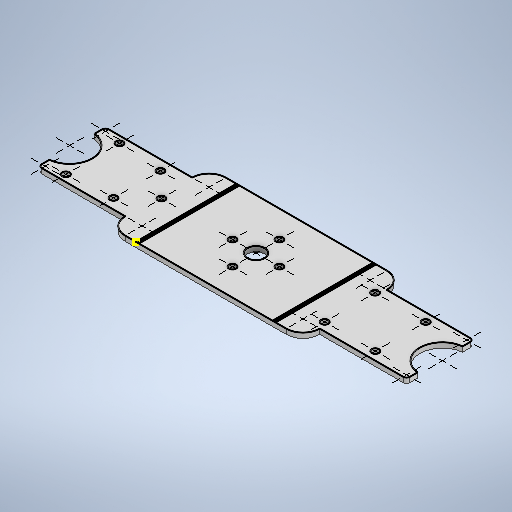
# Autodesk Inventor part: axis_13_top_frame
Saved by Autodesk Inventor 2026.1 (Build 301233000, 233)
## iProperties
Created: 2025-08-22
Part Number: axis_13_top_frame
Material: Generic
Document SubType Name: Modeling
Designer: LG
Density: 1 g/cm^3
Appearance: Default
Author: LG
Autodesk Inventor part; units mm, degrees
ref_plane "YZ Plane" through (0, 0, 0) normal (1, 0, 0) x (0, 1, 0)
ref_plane "XZ Plane" through (0, 0, 0) normal (0, 1, 0) x (-1, 0, 0)
ref_plane "XY Plane" through (0, 0, 0) normal (0, 0, 1) x (1, 0, 0)
sketch "Sketch1" plane through (0, 0, 0) normal (0, 1, 0) x (-1, 0, 0)
  line L0 (-0.4496, -30) -> (-0.4496, 0)
  line L1 (-41.2289, 0) -> (-41.2289, -30)
  circle A0 centre (-48.8686, -22.525) radius 1.05
  circle A1 centre (-48.8686, -7.475) radius 1.05
  circle A2 centre (-63.9686, -22.525) radius 1.05
  circle A3 centre (-63.9686, -7.475) radius 1.05
  circle A4 centre (27.89, -23) radius 1.05
  circle A5 centre (27.89, -7) radius 1.05
  circle A6 centre (14.67, -22) radius 1.05
  circle A7 centre (14.67, -8) radius 1.05
  circle A8 centre (7.37, -15) radius 1.05
  circle A9 centre (-20.8393, -15) radius 2.6
  circle A10 centre (-27.8393, -15) radius 1.05
  circle A11 centre (-20.8393, -8) radius 1.05
  circle A12 centre (-20.8393, -22) radius 1.05
  circle A13 centre (-13.8393, -15) radius 1.05
  arc A14 (-75.7686, -21.7136) -> (-75.7686, -8.2864) centre (-76.4686, -15) ccw
  line L2 (-75.7686, -24) -> (-75.7686, -21.7136)
  arc A15 (-75.7686, -24) -> (-74.7686, -25) centre (-74.7686, -24) ccw
  line L3 (-74.7686, -25) -> (-49.8686, -25)
  arc A16 (-49.8686, -25) -> (-44.8686, -30) centre (-44.8686, -25) ccw
  line L4 (3.19, -30) -> (-44.8686, -30)
  arc A17 (3.19, -30) -> (8.19, -25) centre (3.19, -25) ccw
  line L5 (8.19, -25) -> (33.09, -25)
  arc A18 (33.09, -25) -> (34.09, -24) centre (33.09, -24) ccw
  line L6 (34.09, -21.7136) -> (34.09, -24)
  arc A19 (34.09, -8.2864) -> (34.09, -21.7136) centre (34.79, -15) ccw
  line L7 (34.09, -6) -> (34.09, -8.2864)
  arc A20 (34.09, -6) -> (33.09, -5) centre (33.09, -6) ccw
  line L8 (33.09, -5) -> (8.19, -5)
  arc A21 (8.19, -5) -> (3.19, 0) centre (3.19, -5) ccw
  line L9 (-44.8686, 0) -> (3.19, 0)
  arc A22 (-44.8686, 0) -> (-49.8686, -5) centre (-44.8686, -5) ccw
  line L10 (-49.8686, -5) -> (-74.7686, -5)
  arc A23 (-74.7686, -5) -> (-75.7686, -6) centre (-74.7686, -6) ccw
  line L11 (-75.7686, -8.2864) -> (-75.7686, -6)
  line L12 (-41.6786, -30) -> (-41.6786, 0)
  line L13 (-40.7793, 0) -> (-40.7793, -30)
  line L14 (-0.8993, -30) -> (-0.8993, 0)
  line L15 (0, 0) -> (0, -30)
  constraints: 32 end point, 24 centre point, 20 point on circle, 19 equal radius, 16 tangent, 12 point on line, 10 vertical, 9 parallel, 6 horizontal, 4 perpendicular, 2 collinear, 81 other
extrude "Extrusion1" add sketch "Sketch1" against normal blind 1.5
body "Solid1"
